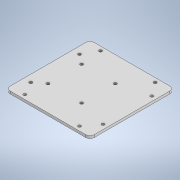
# Autodesk Inventor part: EboxMounting_Plate
Saved by Autodesk Inventor 2021 (Build 250183000, 183)
## iProperties
Created: 2021-10-09
Part Number: EboxMounting_Plate
Material: Generic
Document SubType Name: Modeling
Designer: Jorian Brusind
Density: 1 g/cm^3
Appearance: Default
Author: Jorian Brusind
Autodesk Inventor part; units mm, degrees
ref_plane "YZ Plane" through (0, 0, 0) normal (1, 0, 0) x (0, 1, 0)
ref_plane "XZ Plane" through (0, 0, 0) normal (0, 1, 0) x (-1, 0, 0)
ref_plane "XY Plane" through (0, 0, 0) normal (0, 0, 1) x (1, 0, 0)
sketch "Sketch2" plane through (0, 0, 0) normal (0, 1, 0) x (-1, 0, 0)
  line L0 (0, 0) -> (100, 0)
  line L1 (100, 0) -> (100, -100)
  line L2 (100, -100) -> (0, -100)
  line L3 (0, -100) -> (0, 0)
  circle A0 centre (82.5, -5) radius 1.75
  circle A1 centre (82.5, -95) radius 1.75
  circle A2 centre (17.5, -5) radius 1.75
  circle A3 centre (17.5, -95) radius 1.75
  circle A4 centre (80, -30) radius 1.75
  circle A5 centre (91.5, -21) radius 1.75
  circle A6 centre (91.5, -79) radius 1.75
  circle A7 centre (5.5, -21) radius 1.75
  circle A8 centre (5.5, -79) radius 1.75
  line L4 (50, 0) -> (50, -100)
  circle A9 centre (40, -30) radius 1.75
  circle A10 centre (80, -70) radius 1.75
  circle A11 centre (40, -70) radius 1.75
  dimension "d13" = 100
  dimension "d14" = 100
  dimension "d15" = 3.5
  dimension "d16" = 17.5
  dimension "d17" = 5
  dimension "d20" = 90
  dimension "d23" = 65
  dimension "d26" = 3.5
  dimension "d27" = 20
  dimension "d28" = 30
  dimension "d32" = 3.5
  dimension "d35" = 58
  dimension "d38" = 86
  dimension "d41" = 8.5
  dimension "d42" = 21
  dimension "d51" = 40
  dimension "d54" = 40
  constraints: 12 centre point, 10 end point, 4 horizontal, 3 vertical, 2 midpoint, 2 parallel, 1 perpendicular, 18 other
  measures "d13" distance of L1.end L2.end
  measures "d14" distance of L0.end L1.end
  measures "d15" diameter of A0
  measures "d16" distance from line of L1 A0.centre
  measures "d17" distance from line of L0 A0.centre
  measures "d20" distance of A0.centre A1.centre
  measures "d23" distance of A0.centre A2.centre
  measures "d26" diameter of A4
  measures "d27" distance from line of L1 A4.centre
  measures "d28" distance from line of L0 A4.centre
  measures "d32" diameter of A5
  measures "d35" distance of A5.centre A6.centre
  measures "d38" distance of A5.centre A7.centre
  measures "d41" distance from line of L1 A5.centre
  measures "d42" distance from line of L0 A5.centre
  measures "d51" distance of A4.centre A9.centre
  measures "d54" distance of A4.centre A10.centre
extrude "Extrusion2" add sketch "Sketch2" along normal blind 3
fillet "Fillet2" radius 5 4 edges at (0, 1.5, -100) (-100, 1.5, -100) (0, 1.5, 0) (-100, 1.5, 0)
body "Solid2"
